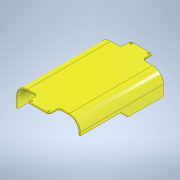
# Autodesk Inventor part: Cover_Superior
Saved by Autodesk Inventor 2020 (Build 240168000, 168)
## iProperties
Created: 2021-06-25
Part Number: Cover_Superior
Material: Plástico PC/ABS
Document SubType Name: Modeling
Designer: JCarlos
Density: 0.357273 g/cm^3
Appearance: Amarelo
Author: JCarlos
Autodesk Inventor part; units mm, degrees
ref_plane "YZ Plane" through (0, 0, 0) normal (1, 0, 0) x (0, 1, 0)
ref_plane "XZ Plane" through (0, 0, 0) normal (0, 1, 0) x (-1, 0, 0)
ref_plane "XY Plane" through (0, 0, 0) normal (0, 0, 1) x (1, 0, 0)
sketch "Esboço1" plane through (0, 0, 0) normal (0, 0, 1) x (1, 0, 0)
  line L0 (42.5, 35) -> (-42.5, 35)
  line L1 (-62.5, 15) -> (-62.5, 0)
  line L2 (62.5, 0) -> (62.5, 15)
  arc A0 (62.5, 15) -> (42.5, 35) centre (42.5, 15) ccw
  arc A1 (-42.5, 35) -> (-62.5, 15) centre (-42.5, 15) ccw
  line L3 (-42.3651, 37) -> (42.5, 37)
  arc A2 (64.5, 15) -> (42.5, 37) centre (42.5, 15) ccw
  line L4 (64.5, 15) -> (64.5, 0)
  line L5 (-64.5004, 0) -> (-64.5004, 15)
  line L6 (-64.5004, 0) -> (-62.5, 0)
  line L7 (62.5, 0) -> (64.5, 0)
  arc A3 (-42.3651, 37) -> (-64.5004, 15) centre (-42.5, 15) ccw
  point P0 (0, 0)
  point P1 (0, 0)
  point P2 (0, 35)
  point P3 (-63.5002, 0)
  dimension "d3" = 20
  dimension "d21" = 2
  dimension "d22" = 37
  dimension "d23" = 125
  dimension "d24" = 2.0004
  dimension "d25" = 2
  dimension "d27" = 2
  dimension "d49" = 2.0004
  constraints: 16 end point, 8 point on circle, 5 tangent, 4 centre point, 2 horizontal alignment, 2 midpoint, 2 parallel, 2 perpendicular, 1 coincident, 1 collinear, 1 concentric, 1 equal radius, 1 vertical alignment, 1 other
  measures "d3" radius of A0
  measures "d21" distance between parallel lines of L0 L3
  measures "d22" distance between parallel lines of L3 L6
  measures "d23" distance between parallel lines of L2 L1
  measures "d24" distance between parallel lines of L1 L5
  measures "d25" distance between parallel lines of L2 L4
  measures "d27" radial gap between concentric circles of A0 A2
  measures "d49" radial gap between concentric circles of A1 A3
extrude "Extrusão1" add sketch "Esboço1" along normal mid plane 170
sketch "Esboço2" plane through (64.5, 0, 85) normal (1, 0, 0) x (0, 0, -1)
  line L0 (170, 0) -> (0, 0) projected
  line L1 (170, 0) -> (170, -7.5)
  line L2 (170, -7.5) -> (99.2426, -7.5)
  line L3 (97.1213, -6.6213) -> (83.8787, 6.6213)
  line L4 (81.7574, 7.5) -> (0, 7.5)
  line L5 (0, 0) -> (0, 15) projected
  line L6 (170, 15) -> (170, 0) projected
  line L7 (170, 0) -> (0, 0)
  line L8 (0, 0) -> (0, 7.5)
  arc A0 (83.8787, 6.6213) -> (81.7574, 7.5) centre (81.7574, 4.5) ccw
  arc A1 (97.1213, -6.6213) -> (99.2426, -7.5) centre (99.2426, -4.5) ccw
  point P0 (85, 0)
  point P1 (98, -7.5)
  point P2 (83, 7.5)
  point P3 (90.5, 0)
  point P4 (90.5, 0)
  dimension "d31" = 7.5
  dimension "d32" = 135
  dimension "d33" = 7.5
  dimension "d34" = 72
  dimension "d35" = 83
  dimension "d40" = 3
  constraints: 12 end point, 4 point on circle, 4 point on line, 4 tangent, 2 centre point, 2 perpendicular, 1 collinear, 1 equal radius, 1 midpoint, 1 parallel, 1 vertical
  measures "d31" distance between parallel lines of L0 L2
  measures "d32" angle of L2 L3
  measures "d33" distance between parallel lines of L0 L4
  measures "d34" distance from line of point (98, -7.5) L6
  measures "d35" distance from line of point (83, 7.5) L5
  measures "d40" radius of A0
extrude "Extrusão2" add sketch "Esboço2" against normal blind 2 contours L1 L2 A1 L3 L0
extrude "Extrusão3" cut sketch "Esboço2" against normal blind 2 contours L0 L5 L4 A0 L3
sketch "Esboço3" plane through (-64.5004, 0, 85) normal (-1, 0, 0) x (0, 0, 1)
  line L0 (-170, 0) -> (0, 0) projected
  line L1 (0, 0) -> (0, -7.5)
  line L2 (0, -7.5) -> (-70.7574, -7.5)
  line L3 (-72.8787, -6.6213) -> (-86.1213, 6.6213)
  line L4 (-88.2426, 7.5) -> (-170, 7.5)
  line L5 (-170, 7.5) -> (-170, 0)
  line L6 (-170, 15) -> (-170, -7.5) projected
  line L7 (0, 0) -> (-170, 0)
  line L8 (-170, 0) -> (0, 0) projected
  arc A0 (-86.1213, 6.6213) -> (-88.2426, 7.5) centre (-88.2426, 4.5) ccw
  arc A1 (-72.8787, -6.6213) -> (-70.7574, -7.5) centre (-70.7574, -4.5) ccw
  point P0 (-85, 0)
  point P1 (-72, -7.5)
  point P2 (-87, 7.5)
  point P3 (-79.5, 0)
  point P4 (-170, 0)
  point P5 (-79.5, 0)
  dimension "d41" = 7.5
  dimension "d42" = 72
  dimension "d43" = 135
  dimension "d50" = 3
  dimension "d61" = 7.5
  constraints: 12 end point, 5 point on line, 4 point on circle, 4 tangent, 3 perpendicular, 2 centre point, 2 parallel, 1 equal radius, 1 vertical
  measures "d41" distance between parallel lines of L2 L0
  measures "d42" distance from line of point (-72, -7.5) L1
  measures "d43" angle of L2 L3
  measures "d50" radius of A0
  measures "d61" distance of L4.end L5.end
extrude "Extrusão4" add sketch "Esboço3" against normal up to surface (2.0004 mm away) contours L0 L1 L2 A1 L3
extrude "Extrusão5" cut sketch "Esboço3" against normal up to surface (2.0004 mm away) contours L5 L4 A0 L3 L0
sketch "Esboço4" plane through (-42.3651, 37, 85) normal (0, 1, 0) x (1, 0, 0)
  line L0 (84.8651, 0) -> (0, 0) projected
  line L1 (64.8651, 0) -> (19.8651, 0)
  line L2 (19.8651, 0) -> (19.8651, -20)
  line L3 (19.8651, -20) -> (64.8651, -20)
  line L4 (64.8651, -20) -> (64.8651, 0)
  point P0 (42.3651, 85)
  point P1 (42.3651, -20)
  dimension "d51" = 20
  dimension "d52" = 45
  constraints: 8 end point, 2 parallel, 1 horizontal, 1 midpoint, 1 perpendicular, 1 point on line, 1 vertical alignment
  measures "d51" distance of L3.end L1.start
  measures "d52" distance of L2.end L3.end
extrude "Extrusão6" add sketch "Esboço4" against normal blind 2
sketch "Esboço5" plane through (-42.3651, 37, -85) normal (0, 1, 0) x (1, 0, 0)
  circle A0 centre (24.8651, -185.5) radius 1.75 projected
  circle A1 centre (59.8651, -185.5) radius 1.75 projected
  point P0 (42.3651, -85)
extrude "Extrusão7" cut sketch "Esboço5" against normal through all
mirror "Espelhamento1" about plane through (0, 0, 0) normal (0, 0, 1) of "Extrusão6", "Extrusão7"
fillet "Arredondamento2" radius 5 8 edges at (22.5, 36, 105) (22.5, 36, 85) (-22.5, 36, 105) (-22.5, 36, 85) (22.5, 36, -85) (22.5, 36, -105) (-22.5, 36, -105) (-22.5, 36, -85)
fillet "Arredondamento3" radius 2.5 4 edges at (63.5, 7.5, 85) (-63.5002, -7.5, 85) (63.5, -7.5, -85) (-63.5002, 7.5, -85)
fillet "Arredondamento4" radius 1 40 edges at (-23.9645, 37, 86.4645) (-22.5, 37, 95) (-21.0355, 37, 103.5355) (0, 37, 105) (21.0355, 37, 103.5355) (22.5, 37, 95) (23.9645, 37, 86.4645) (35, 37, 85) (58.0563, 30.5563, 85) (64.5, 12.5, 85) (64.5, 8.2322, 84.2678) (64.5, 7.5, 42.8713) (64.5, 7.2716, 2.0946) (64.5, 0, -5.5) (64.5, -7.2716, -13.0946) (64.5, -7.5, -48.3713) (64.5, -6.7678, -84.2678) (64.5, 5, -85) (58.0563, 30.5563, -85) (35, 37, -85) (23.9645, 37, -86.4645) (22.5, 37, -95) (21.0355, 37, -103.5355) (0, 37, -105) (-21.0355, 37, -103.5355) (-22.5, 37, -95) (-23.9645, 37, -86.4645) (-34.9326, 37, -85) (-34.9326, 37, 85) (-64.5004, 5, 85) (-64.5004, -6.7678, 84.2678) (-64.5004, -7.5, 48.3713) (-64.5004, -7.2716, 13.0946) (-64.5004, 0, 5.5) (-64.5004, 7.2716, -2.0946) (-64.5004, 7.5, -42.8713) (-64.5004, 8.2322, -84.2678) (-64.5004, 12.5, -85) (-58.0089, 30.6042, -85) (-58.0089, 30.6042, 85)
equation "\"d33\" = d31"
equation "\"d61\" = d41"
